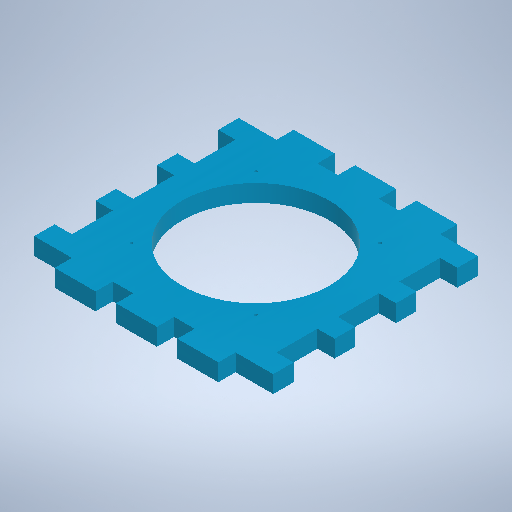
# Autodesk Inventor part: 2
Saved by Autodesk Inventor 2025.3 (Build 293356000, 356)
## iProperties
Created: 2025-12-22
Part Number: 2
Material: Generic
Document SubType Name: Sheet Metal
Designer: Balint
Density: 1 g/cm^3
Flat Pattern Width: 25 cm
Flat Pattern Length: 25 cm
Flat Pattern Area: 625 cm^2
Sheet Metal Rule: Default_mm
Sheet Metal Width: 250.000 mm
Sheet Metal Length: 250.000 mm
Sheet Metal Area: 62500.000 mm^2
Appearance: Default
Author: Balint
Autodesk Inventor part; units mm, degrees
ref_plane "YZ Plane" through (0, 0, 0) normal (1, 0, 0) x (0, 1, 0)
ref_plane "XZ Plane" through (0, 0, 0) normal (0, 1, 0) x (-1, 0, 0)
ref_plane "XY Plane" through (0, 0, 0) normal (0, 0, 1) x (1, 0, 0)
sketch "Sketch1" plane through (0, 0, 0) normal (0, 1, 0) x (-1, 0, 0)
  line L0 (-127.7724, 127.5062) -> (122.2276, 127.5062)
  line L1 (122.2276, 127.5062) -> (122.2276, -122.4938)
  line L2 (122.2276, -122.4938) -> (-127.7724, -122.4938)
  line L3 (-127.7724, -122.4938) -> (-127.7724, 127.5062)
  line L4 (104.2276, -104.4938) -> (104.2276, 109.5062)
  line L5 (104.2276, -104.4938) -> (-109.7724, -104.4938)
  line L6 (-109.7724, -104.4938) -> (104.2276, -104.4938)
  line L7 (122.2276, 109.5062) -> (122.2276, 88.1062)
  line L8 (122.2276, 88.1062) -> (104.2276, 88.1062)
  line L9 (104.2276, 88.1062) -> (104.2276, 109.5062)
  line L10 (122.2276, 45.3062) -> (104.2276, 45.3062)
  line L11 (104.2276, 45.3062) -> (104.2276, 23.9062)
  line L12 (104.2276, 23.9062) -> (122.2276, 23.9062)
  line L13 (104.2276, -18.8938) -> (122.2276, -18.8938)
  line L14 (122.2276, -40.2938) -> (104.2276, -40.2938)
  line L15 (122.2276, -83.0938) -> (104.2276, -83.0938)
  line L16 (-127.7724, 127.5062) -> (-127.7724, 109.5062)
  line L17 (104.2276, 109.5062) -> (104.2276, 127.5062)
  line L18 (-127.7724, -83.0938) -> (-109.7724, -83.0938)
  line L19 (-127.7724, -40.2938) -> (-109.7724, -40.2938)
  line L20 (-109.7724, -18.8938) -> (-127.7724, -18.8938)
  line L21 (-109.7724, 23.9062) -> (-127.7724, 23.9062)
  line L22 (-127.7724, 45.3062) -> (-109.7724, 45.3062)
  line L23 (-127.7724, 88.1062) -> (-109.7724, 88.1062)
  line L24 (18.6276, -104.4938) -> (18.6276, -122.4938)
  line L25 (-24.1724, -104.4938) -> (-24.1724, -122.4938)
  line L26 (-45.5724, -122.4938) -> (-45.5724, -104.4938)
  line L27 (-88.3724, -122.4938) -> (-88.3724, -104.4938)
  line L28 (40.0276, -122.4938) -> (40.0276, -104.4938)
  line L29 (82.8276, -122.4938) -> (82.8276, -104.4938)
  line L30 (18.6276, 127.5062) -> (18.6276, 109.5062)
  line L31 (40.0276, 109.5062) -> (40.0276, 127.5062)
  line L32 (82.8276, 109.5062) -> (82.8276, 127.5062)
  line L33 (-45.5724, 109.5062) -> (-45.5724, 127.5062)
  line L34 (-88.3724, 109.5062) -> (-88.3724, 127.5062)
  line L35 (-24.1724, 127.5062) -> (-24.1724, 109.5062)
  line L36 (104.2276, 109.5062) -> (-109.7724, 109.5062)
  line L37 (-109.7724, 109.5062) -> (-109.7724, -104.4938)
  line L38 (-109.7724, 109.5062) -> (-127.7724, 109.5062)
  line L39 (-127.7724, 109.5062) -> (-127.7724, 127.5062)
  line L40 (-127.7724, 127.5062) -> (-109.7724, 127.5062)
  line L41 (-109.7724, 127.5062) -> (-109.7724, 109.5062)
  line L42 (-109.7724, -104.4938) -> (-127.7724, -104.4938)
  line L43 (-127.7724, -104.4938) -> (-127.7724, -122.4938)
  line L44 (-127.7724, -122.4938) -> (-109.7724, -122.4938)
  line L45 (-109.7724, -122.4938) -> (-109.7724, -104.4938)
  line L46 (104.2276, -104.4938) -> (122.2276, -104.4938)
  line L47 (122.2276, -104.4938) -> (122.2276, -122.4938)
  line L48 (122.2276, -122.4938) -> (104.2276, -122.4938)
  line L49 (104.2276, -122.4938) -> (104.2276, -104.4938)
  line L50 (104.2276, 109.5062) -> (122.2276, 109.5062)
  line L51 (122.2276, 109.5062) -> (122.2276, 127.5062)
  line L52 (122.2276, 127.5062) -> (104.2276, 127.5062)
  line L53 (104.2276, 127.5062) -> (104.2276, 109.5062)
  point P0 (0, 0)
  point P1 (-127.7724, -18.8938)
  point P2 (-109.7724, -104.4938)
  point P3 (-109.7724, -104.4938)
  dimension "d0" = 250
  dimension "d1" = 250
  dimension "d2" = 21.4
  measures "d0" distance of L1.end L2.end
  measures "d1" distance of L0.end L1.end
  measures "d2" distance of L7.start L7.end
extrude "Plate1" add sketch "Sketch1" along normal blind 18 contours L38 L37 L23 L3 | L0 L33 L36 L34 | L36 L4 L5 L37 | L22 L37 L21 L3 | L0 L30 L36 L35 | L20 L37 L19 L3 | L0 L32 L36 L31 | L18 L37 L42 L3 | L50 L1 L8 L4 | L5 L26 L2 L27 | L10 L1 L12 L4 | L5 L24 L2 L25 | L13 L1 L14 L4 | L5 L29 L2 L28 | L15 L1 L46 L4
sketch "Sketch2" plane through (0, 18, 0) normal (0, 1, 0) x (1, 0, 0)
  circle A0 centre (0, 0) radius 77.1
  line L0 (-65, 65) -> (65, 65)
  line L1 (65, 65) -> (65, -65)
  line L2 (65, -65) -> (-65, -65)
  line L3 (-65, -65) -> (-65, 65)
  line L4 (-65, 65) -> (65, -65) construction
  line L5 (65, 65) -> (-65, -65) construction
  circle A1 centre (65, 65) radius 1.5
  circle A2 centre (65, -65) radius 1.5
  circle A3 centre (-65, -65) radius 1.5
  circle A4 centre (-65, 65) radius 1.5
  dimension "d4" = 154.2
  dimension "d5" = 130
  dimension "d6" = 130
  dimension "d7" = 3
  dimension "d8" = 3
  dimension "d9" = 3
  dimension "d10" = 3
  constraints: 12 end point, 5 centre point, 5 coincident, 2 midpoint, 2 parallel, 1 horizontal, 1 perpendicular
  measures "d4" diameter of A0
  measures "d5" distance of L1.end L2.end
  measures "d6" distance of L0.end L1.end
  measures "d7" diameter of A1
  measures "d8" diameter of A2
  measures "d9" diameter of A3
  measures "d10" diameter of A4
extrude "Cut1" cut sketch "Sketch2" against normal blind 18 contours A0 L1 | L1 A0 L2 L3 L0 | L0 A0 | A1 L0 L1 | L1 L0 A1 | A0 L2 | A2 L2 L1 | L1 L2 A2 | L3 A0 | A4 L3 L0 | L0 L3 A4 | A3 L3 L2 | L2 L3 A3
equation "\"d11\" = Thickness"
equation "\"d3\" = Thickness"
equation "\"BendRadius\" = Thickness"
equation "\"BendReliefWidth\" = Thickness"
equation "\"BendReliefDepth\" = 0.5 * Thickness"
equation "\"CornerReliefSize\" = 4 * Thickness"
equation "\"MinimumRemnant\" = 2 * Thickness"
equation "\"TransitionRadius\" = BendRadius"
equation "\"JacobiRadiusSize\" = BendRadius"
equation "\"GapSize\" = Thickness"
equation "\"Thickness\" = 18"
body "Solid1"
